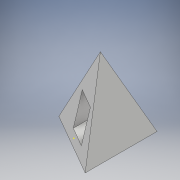
# Autodesk Inventor part: ДЗ2 Курганова
Saved by Autodesk Inventor 2017 (Build 210142000, 142)
## iProperties
Part Number: ДЗ2 Курганова
Material: Типовые
Document SubType Name: Modeling
Designer: Sasha
Density: 1 g/cm^3
Appearance: По умолчанию
Mass: 47.791 g
Surface Area: 131.841 cm^2
Volume: 47.791 cm^3
Author: Sasha
Autodesk Inventor part; units mm, degrees
ref_plane "YZ Plane" through (0, 0, 0) normal (1, 0, 0) x (0, 1, 0)
ref_plane "XZ Plane" through (0, 0, 0) normal (0, 1, 0) x (-1, 0, 0)
sketch "Эскиз1" plane through (0, 0, 0) normal (0, 0, 1) x (1, 0, 0)
  line L0 (-43.3013, 0) -> (21.6506, 37.5)
  line L1 (21.6506, 37.5) -> (21.6506, -37.5)
  line L2 (21.6506, -37.5) -> (-43.3013, 0)
  point P0 (0, 0)
  point P1 (0, 0)
  dimension "d2" = 75
  constraints: 6 end point, 1 coincident, 7 other
  measures "d2" distance of L0.end L1.end
ref_plane "РабПлоскость1" through (0, 0, 80) normal (0, 0, 1) x (1, 0, 0)
sketch "Эскиз2" plane through (0, 0, 80) normal (0, 0, 1) x (1, 0, 0)
  point P0 (0, 0)
  point P1 (0, 0)
  constraints: 1 coincident
loft "Лофт1" add profiles "Эскиз1" section 2 point at (0, 0, 80)
sketch "Эскиз3" plane through (0, 0, 0) normal (0, 1, 0) x (-1, 0, 0)
  point P0 (0, 0)
sketch "Эскиз4" plane through (0, 0, 0) normal (0, 1, 0) x (-1, 0, 0)
  line L0 (-5, 10) -> (15, 10)
  line L1 (15, 10) -> (15, 40)
  line L2 (15, 40) -> (-5, 40)
  line L3 (-5, 40) -> (-5, 10)
  line L4 (-5, 10) -> (15, 40) construction
  line L5 (15, 10) -> (-5, 40) construction
  point P0 (0, 0)
  point P1 (0, 0)
  point P2 (5, 25)
  dimension "d8" = 20
  dimension "d9" = 30
  dimension "d10" = 15
  dimension "d12" = 10
  constraints: 12 end point, 2 midpoint, 2 parallel, 1 horizontal, 1 perpendicular
  measures "d8" distance of L1.end L2.end
  measures "d9" distance of L0.end L1.end
  measures "d10" distance from line of point (0, 0) L1
  measures "d12" distance from line of point (0, 0) L0
extrude "Выдавливание1" cut sketch "Эскиз4" along normal through all both and the other way through all
sketch "Эскиз5" plane through (21.6506, -37.5, 0) normal (-0.4826376, -0.8359528, 0.2612353) x (0.8428609, -0.3622752, 0.3979224)
  point P0 (-31.8338, 20.6119)
